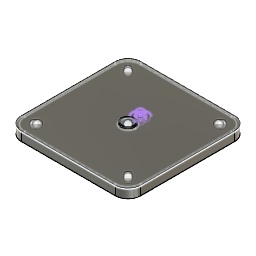
TeleRad_Assembly (Autodesk Fusion 360 archive; units mm, degrees)
design "BasePlate"
part number: 2026-04-09-20-58-55-173
Autodesk Fusion 360 part; units mm, degrees
sketch "Sketch4" plane through (0, 0, 0) normal (0, 0, 1) x (1, 0, 0)
  line L0 (75, 0) -> (625, 0)
  line L1 (700, 75) -> (700, 625)
  line L2 (625, 700) -> (75, 700)
  line L3 (0, 625) -> (0, 75)
  arc A0 (0, 75) -> (75, 0) centre (75, 75) ccw
  arc A1 (75, 700) -> (0, 625) centre (75, 625) ccw
  arc A2 (700, 625) -> (625, 700) centre (625, 625) ccw
  arc A3 (625, 0) -> (700, 75) centre (625, 75) ccw
  circle A4 centre (350, 350) radius 34
  circle A5 centre (350, 422.75) radius 11.25
  circle A6 centre (365.5, 407.25) radius 1.55
  circle A7 centre (334.5, 407.25) radius 1.55
  circle A8 centre (334.5, 438.25) radius 1.55
  circle A9 centre (365.5, 438.25) radius 1.55
  point P0 (700, 0)
  point P1 (0, 700)
  dimension "d5" = 700
  dimension "d6" = 700
  dimension "d7" = 75
  dimension "d8" = 75
  dimension "d9" = 75
  dimension "d10" = 75
  dimension "d11" = 68
  dimension "d12" = 350
  dimension "d13" = 350
  dimension "d51" = 22.5
  dimension "d52" = 72.75
  dimension "d53" = 350
  dimension "d54" = 3.1
  dimension "d55" = 15.5
  dimension "d56" = 15.5
  dimension "d58" = 15.5
  dimension "d59" = 15.5
  dimension "d60" = 15.5
  dimension "d61" = 15.5
  dimension "d62" = 15.5
  dimension "d63" = 15.5
  dimension "d64" = 3.1
  dimension "d65" = 3.1
  dimension "d66" = 3.1
  constraint horizontal L0
  constraint vertical L1
  constraint horizontal L2
  constraint vertical L3
  constraint coincident origin L0
  constraint coincident origin L3
  constraint tangent L0 A0
  constraint tangent L3 A0
  constraint coincident P1 L2
  constraint coincident P1 L3
  constraint tangent L2 A1
  constraint tangent L3 A1
  constraint tangent L1 A2
  constraint tangent L2 A2
  constraint coincident P0 L0
  constraint coincident P0 L1
  constraint tangent L0 A3
  constraint tangent L1 A3
  measures "d5" distance of origin P1
  measures "d6" distance of origin P0
  measures "d7" radius of A0
  measures "d8" radius of A1
  measures "d9" radius of A2
  measures "d10" radius of A3
  measures "d11" diameter of A4
  measures "d12" distance of L0 A4.centre
  measures "d13" distance of L3 A4.centre
  measures "d51" diameter of A5
  measures "d52" vertical distance of A4.centre A5.centre
  measures "d53" distance of L3 A5.centre
  measures "d54" diameter of A6
  measures "d55" vertical distance of A5.centre A6.centre
  measures "d56" horizontal distance of A5.centre A6.centre
  measures "d58" horizontal distance of A5.centre A7.centre
  measures "d59" vertical distance of A5.centre A7.centre
  measures "d60" horizontal distance of A5.centre A8.centre
  measures "d61" vertical distance of A5.centre A8.centre
  measures "d62" horizontal distance of A5.centre A9.centre
  measures "d63" vertical distance of A5.centre A9.centre
  measures "d64" diameter of A7
  measures "d65" diameter of A8
  measures "d66" diameter of A9
extrude "Extrude2" add sketch "Sketch4" along normal blind 5
sketch "Sketch5" plane through (0, 0, 0) normal (0, 0, -1) x (1, 0, 0)
  circle A0 centre (350, -350) radius 34
  arc A1 (700, -75) -> (625, 0) centre (625, -75) ccw
  line L0 (625, 0) -> (75, 0)
  arc A2 (75, 0) -> (0, -75) centre (75, -75) ccw
  line L1 (0, -75) -> (0, -625)
  arc A3 (0, -625) -> (75, -700) centre (75, -625) ccw
  line L2 (75, -700) -> (625, -700)
  arc A4 (625, -700) -> (700, -625) centre (625, -625) ccw
  line L3 (700, -625) -> (700, -75)
  line L4 (625, -700) -> (75, -700)
  line L5 (0, -625) -> (0, -75)
  line L6 (75, 0) -> (625, 0)
  line L7 (700, -75) -> (700, -625)
  arc A5 (625, -700) -> (700, -625) centre (625, -625) ccw
  arc A6 (0, -625) -> (75, -700) centre (75, -625) ccw
  arc A7 (75, 0) -> (0, -75) centre (75, -75) ccw
  arc A8 (700, -75) -> (625, 0) centre (625, -75) ccw
  line L8 (615, -690) -> (85, -690)
  line L9 (10, -615) -> (10, -85)
  line L10 (85, -10) -> (615, -10)
  line L11 (690, -85) -> (690, -615)
  arc A9 (615, -690) -> (690, -615) centre (615, -615) ccw
  arc A10 (10, -615) -> (85, -690) centre (85, -615) ccw
  arc A11 (85, -10) -> (10, -85) centre (85, -85) ccw
  arc A12 (690, -85) -> (615, -10) centre (615, -85) ccw
  circle A13 centre (350, -350) radius 44
  circle A14 centre (350, -422.75) radius 11.25
  circle A15 centre (334.5, -407.25) radius 1.55
  circle A16 centre (365.5, -438.25) radius 1.55
  circle A17 centre (365.5, -407.25) radius 1.55
  circle A18 centre (334.5, -438.25) radius 1.55
  dimension "d32" = 75
  dimension "d33" = 75
  dimension "d34" = 75
  dimension "d35" = 75
  dimension "d36" = 75
  dimension "d37" = 75
  dimension "d38" = 75
  dimension "d39" = 75
  dimension "d40" = 10
  dimension "d41" = 10
  dimension "d42" = 10
  dimension "d43" = 10
  dimension "d46" = 10
  constraint horizontal L4
  constraint vertical L5
  constraint horizontal L6
  constraint vertical L7
  constraint tangent L4 A5
  constraint tangent L7 A5
  constraint tangent L4 A6
  constraint tangent L5 A6
  constraint tangent L5 A7
  constraint tangent L6 A7
  constraint tangent L6 A8
  constraint tangent L7 A8
  constraint horizontal L8
  constraint vertical L9
  constraint horizontal L10
  constraint vertical L11
  constraint tangent L8 A9
  constraint tangent L11 A9
  constraint tangent L8 A10
  constraint tangent L9 A10
  constraint tangent L9 A11
  constraint tangent L10 A11
  constraint tangent L10 A12
  constraint tangent L11 A12
  constraint collinear L1 L5
  constraint collinear L2 L4
  constraint collinear L3 L7
  constraint collinear L0 L6
  measures "d32" radius of A5
  measures "d33" radius of A6
  measures "d34" radius of A7
  measures "d35" radius of A8
  measures "d36" radius of A9
  measures "d37" radius of A10
  measures "d38" radius of A11
  measures "d39" radius of A12
  measures "d40" distance of L4 L8
  measures "d41" distance of L6 L10
  measures "d42" distance of L5 L9
  measures "d43" distance of L7 L11
extrude "Extrude3" add sketch "Sketch5" along normal blind 50 contours A1 L0 A2 L1 A3 L2 A4 L3 L4 L5 L6 L7 A5 A6 A7 A8
extrude "Extrude4" add sketch "Sketch5" along normal blind 15 contours A13
extrude "Extrude5" add 1 faces at (390.3763, 353.8751, -15) along direction (0, 0, -1) blind 35
sketch "Sketch6" plane through (0, 0, 5) normal (0, 0, 1) x (-1, 0, 0)
  circle A0 centre (-365.5, -438.25) radius 1.55
  circle A1 centre (-350, -350) radius 34
  circle A2 centre (-334.5, -438.25) radius 1.55
  circle A3 centre (-350, -422.75) radius 11.25
  circle A4 centre (-365.5, -407.25) radius 1.55
  circle A5 centre (-334.5, -407.25) radius 1.55
  arc A6 (-625, 0) -> (-700, -75) centre (-625, -75) ccw
  line L0 (-700, -75) -> (-700, -625)
  arc A7 (-700, -625) -> (-625, -700) centre (-625, -625) ccw
  line L1 (-625, -700) -> (-75, -700)
  arc A8 (-75, -700) -> (0, -625) centre (-75, -625) ccw
  line L2 (0, -625) -> (0, -75)
  arc A9 (0, -75) -> (-75, 0) centre (-75, -75) ccw
  line L3 (-75, 0) -> (-625, 0)
  circle A10 centre (-350, -350) radius 39
  dimension "d67" = 5
extrude "Extrude6" add sketch "Sketch6" along normal blind 7.5 contours A10
equation "d49 = 55 mm - 20 mm"
equation "d55 = ( 31 / 2 ) * 1 mm"
equation "d56 = ( 31 / 2 ) * 1 mm"
equation "d58 = ( 31 / 2 ) * 1 mm"
equation "d59 = ( 31 / 2 ) * 1 mm"
equation "d60 = ( 31 / 2 ) * 1 mm"
equation "d61 = ( 31 / 2 ) * 1 mm"
equation "d62 = ( 31 / 2 ) * 1 mm"
equation "d63 = ( 31 / 2 ) * 1 mm"
named bodies: "Baseplate"

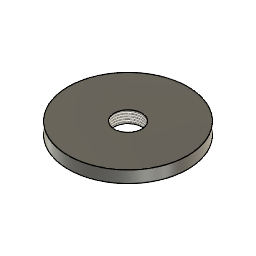
design "Altitude Counterweight Thread"
part number: 2026-04-14-15-13-28-542
Autodesk Fusion 360 part; units mm, degrees
sketch "Sketch1" plane through (0, 0, 0) normal (0, 0, 1) x (1, 0, 0)
  circle A0 centre (0, 0) radius 50
  dimension "d1" = 100
  constraint coincident A0.centre origin
  measures "d1" diameter of A0
extrude "Extrude1" add sketch "Sketch1" along normal blind 10
hole "Hole1" at (0, 0, 10) direction (0, 0, -1) diameter 23.022 end through all
thread "Thread1" "ISO Metric profile 25.0 M25x2 M25x2 6H" thread offset 0 thread depth 7.4

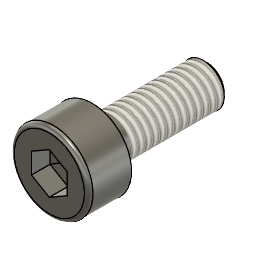
design "8xM3 hexagon head"
description: Hexagon Socket Head Cap Screw ISO 4762 - M3 x 8
part number: ISO 4762 - M3 x 8 Steel 4.6 Plain
Autodesk Fusion 360 part; units mm, degrees
sketch "Sketch1" plane through (0, 0, 0) normal (0, 1, 0) x (1, 0, 0)
  line L0 (-1.5, 0) -> (-1.5, 8)
  line L1 (-1.5, 8) -> (0, 8)
  line L2 (0, 8) -> (0, -3)
  line L3 (-1.5, 0) -> (-2.75, 0)
  line L4 (-2.75, 0) -> (-2.75, -3)
  line L5 (-2.75, -3) -> (0, -3)
  dimension "d9" = 3
  dimension "d106" = 3
  dimension "d107" = 8
  dimension "d116" = 5.5
  constraint perpendicular L0 L1
  constraint collinear origin L1.end L2.end
  constraint perpendicular L0 L3
  constraint coincident origin L3
  constraint vertical L2
  constraint coincident L2 L5.end
  constraint perpendicular L2 L5
  measures "d106" distance of L3 L5
  measures "d107" distance of origin L1
revolve "Revolve1" add sketch "Sketch1" angle 360 about axis through (0, 0, -8) along (0, 0, 1)
ref_plane "WorkPlane1" through (0, 0, 3) normal (0, 0, 1) x (1, 0, 0)
sketch "Sketch6" plane through (0, 0, 3) normal (0, 0, 1) x (1, 0, 0)
  line L0 (-1.25, 0.7217) -> (-1.25, -0.7217)
  line L1 (-1.25, -0.7217) -> (0, -1.4434)
  line L2 (0, -1.4434) -> (1.25, -0.7217)
  line L3 (1.25, -0.7217) -> (1.25, 0.7217)
  line L4 (1.25, 0.7217) -> (0, 1.4434)
  line L5 (0, 1.4434) -> (-1.25, 0.7217)
  dimension "d117" = 2.5
  constraint vertical L0
  measures "d117" distance of L0 L3
extrude "Extrude1" cut sketch "Sketch6" against normal blind 1.3
extrude "Extrude2" cut 1 faces at (0.4167, -0.2406, 1.7) along direction (0, 0, -1) blind 1.3 draft -85
fillet "Fillet4" radius 0.3 1 edges at (-2.5639, 0.9944, 3)
thread "Thread3" "ISO Metric profile 3.0 M3x0.5 M3x0.5 6g" major diameter 2.927 minor diameter 2.3555 pitch 0.5 angle 60 resizes the face on face at (-1.4925, 0.1494, -5.3333) from (0, 0, -1.25) to (0, 0, -8)
sketch "Sketch7" plane through (0, 0, 0) normal (0, 1, 0) x (1, 0, 0)
  line L0 (-1.53, 8) -> (-1.53, 7.7)
  line L1 (-1.53, 7.7) -> (-1.23, 8)
  line L2 (0, 8) -> (0, -3)
  line L3 (-1.53, 8) -> (0, 8)
  dimension "d101" = 45
  dimension "d112" = 0.3
  dimension "d113" = 1.53
  constraint coincident L2.start L3.end
  constraint perpendicular L2 L3
  constraint coincident L1.end L3
  constraint perpendicular L0 L3
  measures "d101" angle of L0 L1
  measures "d112" distance of L0.end L3
  measures "d113" distance of L0 L2.start
revolve "Revolve3" cut sketch "Sketch7" angle 360 about axis through (0, 0, 1.75) along (0, 0, 1)
equation "d9 = adsk_nomdia"
equation "adsk_nomlen = 8.00 mm"
equation "adsk_headh = 3.00 mm"
equation "adsk_headdia = 5.50 mm"
equation "adsk_nomdia = 3.00 mm"
equation "adsk_philwidth = 2.50 mm"
equation "d31 = -adsk_phildepth"
equation "adsk_phildepth = 1.30 mm"
equation "d71 = adsk_headh"
equation "d76 = -adsk_phildepth"
equation "adsk_thrlen = 6.75 mm"
equation "d86 = adsk_nomdia * 0.1"
equation "adsk_startang = 45.00 deg"
equation "d101 = adsk_startang"
equation "adsk_pitch1 = 0.50 mm"
equation "adsk_startlen = 0.30 mm"
equation "d106 = adsk_headh"
equation "d107 = adsk_nomlen"
equation "d112 = adsk_startlen"
equation "d113 = adsk_nomdia * 0.51"
equation "d115 = min(adsk_thrlen; adsk_nomlen - 0.001 mm)"
equation "d116 = adsk_headdia"
equation "d117 = adsk_philwidth"

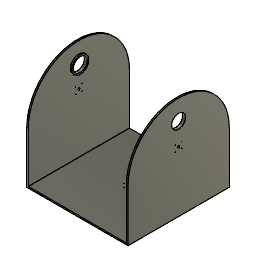
design "Altitude Baseplate"
part number: 2026-04-09-23-56-47-011
Autodesk Fusion 360 part; units mm, degrees
sketch "Sketch1" plane through (0, 0, 0) normal (0, 0, 1) x (1, 0, 0)
  line L0 (0, 0) -> (500, 0)
  line L1 (500, 0) -> (500, 500)
  line L2 (500, 500) -> (0, 500)
  line L3 (0, 500) -> (0, 0)
  circle A0 centre (250, 250) radius 1.5
  circle A1 centre (230, 249.99) radius 1.5
  circle A2 centre (270, 250.01) radius 1.5
  circle A3 centre (249.99, 270) radius 1.5
  circle A4 centre (250.01, 230) radius 1.5
  point P0 (250.01, 230)
  point P1 (270, 250.01)
  point P2 (249.99, 270)
  dimension "d1" = 500
  dimension "d2" = 500
  dimension "d3" = 3
  dimension "d4" = 250
  dimension "d5" = 250
  dimension "d50" = 3
  dimension "d52" = 360
  dimension "d53" = 20
  dimension "d54" = 0.01
  dimension "d55" = 3
  dimension "d56" = 3
  dimension "d57" = 3
  constraint horizontal L0
  constraint vertical L1
  constraint horizontal L2
  constraint vertical L3
  constraint coincident L0.start L3.end
  constraint coincident P1 A2.centre
  constraint coincident P2 A3.centre
  constraint coincident P0 A4.centre
  measures "d1" distance of L1.end L2.end
  measures "d2" distance of L0.start L2.end
  measures "d3" diameter of A0
  measures "d4" distance of L3 A0.centre
  measures "d5" distance of L2 A0.centre
  measures "d50" diameter of A1
  measures "d53" horizontal distance of A0.centre A1.centre
  measures "d54" vertical distance of A0.centre A1.centre
  measures "d55" diameter of A2
  measures "d56" diameter of A3
  measures "d57" diameter of A4
extrude "Extrude1" add sketch "Sketch1" along normal blind 7.5
sketch "Sketch2" plane through (0, 0, 7.5) normal (0, 0, 1) x (-1, 0, 0)
  circle A0 centre (-250, -250) radius 1.5
  line L0 (0, -500) -> (0, 0)
  line L1 (0, 0) -> (-500, 0)
  line L2 (-500, 0) -> (-500, -500)
  line L3 (-500, -500) -> (0, -500)
  line L4 (0, -500) -> (-7.5, -500)
  line L5 (-7.5, -500) -> (-7.5, 0)
  line L6 (-7.5, 0) -> (0, 0)
  line L7 (0, 0) -> (0, -500)
  line L8 (-500, -500) -> (-492.5, -500)
  line L9 (-492.5, -500) -> (-492.5, 0)
  line L10 (-492.5, 0) -> (-500, 0)
  line L11 (-500, 0) -> (-500, -500)
  circle A1 centre (-270, -250.01) radius 1.5
  circle A2 centre (-249.99, -270) radius 1.5
  circle A3 centre (-230, -249.99) radius 1.5
  circle A4 centre (-250.01, -230) radius 1.5
  dimension "d8" = 7.5
  dimension "d9" = 7.5
  constraint horizontal L4
  constraint vertical L5
  constraint horizontal L6
  constraint vertical L7
  constraint coincident L1 L5.end
  constraint coincident L0.start L3.end
  constraint horizontal L8
  constraint vertical L9
  constraint horizontal L10
  constraint vertical L11
  constraint coincident L1 L9.end
  constraint coincident L2.end L3.start
  measures "d8" distance of L5 L7
  measures "d9" distance of L9 L11
extrude "Extrude2" add sketch "Sketch2" along normal blind 500 contours L0 L1 L3 L4 L5 L6 L7 | L1 L2 L3 L8 L9 L10 L11
fillet "Fillet1" radius 250 1 edges at (3.75, 500, 507.5)
fillet "Fillet2" radius 250 1 edges at (3.75, 0, 507.5)
fillet "Fillet3" radius 250 1 edges at (496.25, 500, 507.5)
fillet "Fillet4" radius 250 1 edges at (496.25, 0, 507.5)
sketch "Sketch3" plane through (0, 0, 0) normal (-1, 0, 0) x (0, -1, 0)
  arc A0 (0, 257.5) -> (-500, 257.5) centre (-250, 257.5) ccw
  line L0 (-500, 257.5) -> (-500, 0)
  line L1 (-500, 0) -> (0, 0)
  line L2 (0, 0) -> (0, 257.5)
  circle A1 centre (-250, 407.5) radius 34
  dimension "d20" = 68
  dimension "d22" = 250
  measures "d20" diameter of A1
  measures "d22" distance of L0 A1.centre
hole "Hole1" at (0, 250, 407.5) direction (1, 0, 0) diameter 68 depth 6000 tip angle 118
sketch "Sketch4" plane through (7.5, 0, 0) normal (1, 0, 0) x (0, 1, 0)
  circle A0 centre (250, 407.5) radius 34
  arc A1 (500, 257.5) -> (0, 257.5) centre (250, 257.5) ccw
  line L0 (0, 257.5) -> (0, 7.5)
  line L1 (0, 7.5) -> (500, 7.5)
  line L2 (500, 7.5) -> (500, 257.5)
  circle A2 centre (250, 407.5) radius 41.5
  dimension "d26" = 7.5
extrude "Extrude3" add sketch "Sketch4" along normal blind 7.5 contours A2
sketch "Sketch5" plane through (492.5, 0, 0) normal (-1, 0, 0) x (0, -1, 0)
  circle A0 centre (-250, 407.5) radius 34
  arc A1 (0, 257.5) -> (-500, 257.5) centre (-250, 257.5) ccw
  line L0 (-500, 257.5) -> (-500, 7.5)
  line L1 (-500, 7.5) -> (0, 7.5)
  line L2 (0, 7.5) -> (0, 257.5)
  circle A2 centre (-250, 407.5) radius 41.5
  dimension "d29" = 7.5
extrude "Extrude4" add sketch "Sketch5" along normal blind 7.5 contours A2
sketch "Sketch6" plane through (500, 0, 0) normal (1, 0, 0) x (0, 1, 0)
  circle A0 centre (250, 407.5) radius 34
  arc A1 (500, 257.5) -> (0, 257.5) centre (250, 257.5) ccw
  line L0 (0, 257.5) -> (0, 0)
  line L1 (0, 0) -> (500, 0)
  line L2 (500, 0) -> (500, 257.5)
  circle A2 centre (250, 298.7) radius 5.625
  circle A3 centre (234.5, 314.2) radius 1.55
  circle A4 centre (265.5, 314.2) radius 1.55
  circle A5 centre (265.5, 283.2) radius 1.55
  circle A6 centre (234.5, 283.2) radius 1.55
  dimension "d32" = 11.25
  dimension "d33" = 108.8
  dimension "d37" = 298.7
  dimension "d38" = 15.5
  dimension "d39" = 15.5
  dimension "d40" = 15.5
  dimension "d41" = 15.5
  dimension "d42" = 15.5
  dimension "d43" = 15.5
  dimension "d44" = 15.5
  dimension "d45" = 15.5
  dimension "d46" = 3.1
  dimension "d47" = 3.1
  dimension "d48" = 3.1
  dimension "d49" = 3.1
  measures "d32" diameter of A2
  measures "d33" distance of A0.centre A2.centre
  measures "d37" distance of L1 A2.centre
  measures "d38" vertical distance of A2.centre A6.centre
  measures "d39" horizontal distance of A2.centre A6.centre
  measures "d40" vertical distance of A2.centre A3.centre
  measures "d41" horizontal distance of A2.centre A3.centre
  measures "d42" horizontal distance of A2.centre A4.centre
  measures "d43" vertical distance of A2.centre A4.centre
  measures "d44" vertical distance of A2.centre A5.centre
  measures "d45" horizontal distance of A2.centre A5.centre
  measures "d46" diameter of A3
  measures "d47" diameter of A4
  measures "d48" diameter of A5
  measures "d49" diameter of A6
extrude "Extrude5" cut sketch "Sketch6" against normal blind 700 contours A2 | A3 | A4 | A5 | A6
equation "d37 = 407.5 mm - 108.8 mm"
equation "d38 = ( 31 / 2 ) * 1 mm"
equation "d39 = ( 31 / 2 ) * 1 mm"
equation "d40 = ( 31 / 2 ) * 1 mm"
equation "d41 = ( 31 / 2 ) * 1 mm"
equation "d42 = ( 31 / 2 ) * 1 mm"
equation "d43 = ( 31 / 2 ) * 1 mm"
equation "d44 = ( 31 / 2 ) * 1 mm"
equation "d45 = ( 31 / 2 ) * 1 mm"
